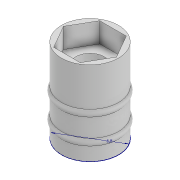
# Autodesk Inventor part: Tuebel
Saved by Autodesk Inventor 2022 (Build 260153000, 153)
## iProperties
Created: 2022-11-28
Part Number: Tuebel
Material: Generisch
Document SubType Name: Modeling
Designer: alexw
Density: 1 g/cm^3
Appearance: Vorgabe
Author: alexw
Autodesk Inventor part; units mm, degrees
ref_plane "YZ Plane" through (0, 0, 0) normal (1, 0, 0) x (0, 1, 0)
ref_plane "XZ Plane" through (0, 0, 0) normal (0, 1, 0) x (-1, 0, 0)
ref_plane "XY Plane" through (0, 0, 0) normal (0, 0, 1) x (1, 0, 0)
sketch "Skizze1" plane through (0, 0, 0) normal (0, 1, 0) x (-1, 0, 0)
  circle A0 centre (0, 0) radius 3.4
  dimension "d0" = 6.8
  constraints: 2 coincident, 1 centre point
  measures "d0" diameter of A0
extrude "Extrusion1" add sketch "Skizze1" along normal blind 10
sketch "Skizze2" plane through (0, 10, 0) normal (0, 1, 0) x (1, 0, 0)
  line L0 (-3.1754, 0) -> (-1.5877, 2.75)
  line L1 (-1.5877, 2.75) -> (1.5877, 2.75)
  line L2 (1.5877, 2.75) -> (3.1754, 0)
  line L3 (3.1754, 0) -> (1.5877, -2.75)
  line L4 (1.5877, -2.75) -> (-1.5877, -2.75)
  line L5 (-1.5877, -2.75) -> (-3.1754, 0)
  line L6 (3.1754, 0) -> (-3.1754, 0) construction
  line L7 (-4.76, 0) -> (4.76, 0) construction
  point P0 (0, 0)
  point P1 (0, 0)
  dimension "d10" = 5.5
  constraints: 14 end point, 1 coincident, 1 collinear, 13 other
  measures "d10" distance between parallel lines of L2 L5
extrude "Extrusion2" cut sketch "Skizze2" against normal blind 2.4
hole "Bohrung2" at (0, 0, 0) direction (0, 1, 0) diameter 3.4 end through all clearance for "Inbusschraube DIN EN ISO 4762" size "M3" standard "DIN"
sketch "Skizze3" plane through (0, 0, 0) normal (1, 0, 0) x (0, 1, 0)
  circle A0 centre (5, 3.1) radius 0.5
  line L0 (10, 2.75) -> (10, 0) projected
  line L1 (0, 0) -> (10, 0) construction
  circle A1 centre (2, 3.1) radius 0.5
  line L2 (2, 3.1) -> (5, 3.1) construction
  line L3 (0, 3.4) -> (10, 3.4) projected
  point P0 (1.6, 3.4)
  point P1 (2.4, 3.4)
  point P2 (4.6, 3.4)
  point P3 (5.4, 3.4)
  dimension "d21" = 3.1
  dimension "d22" = 5
  dimension "d23" = 3
  dimension "d24" = 1
  constraints: 4 end point, 2 centre point, 1 equal radius, 1 horizontal, 1 parallel
  measures "d21" distance from line of L1 L2.end
  measures "d22" horizontal distance of L1.start L2.end
  measures "d23" distance of L2.end L2.start
  measures "d24" diameter of A0
revolve "Umdrehung1" add sketch "Skizze3" angle 360 about axis through (0, 0, 0) along (0, 1, 0) picked at (1.8932, 3.428) picked at (4.8932, 3.428) contours L3 A1 | L3 A0
